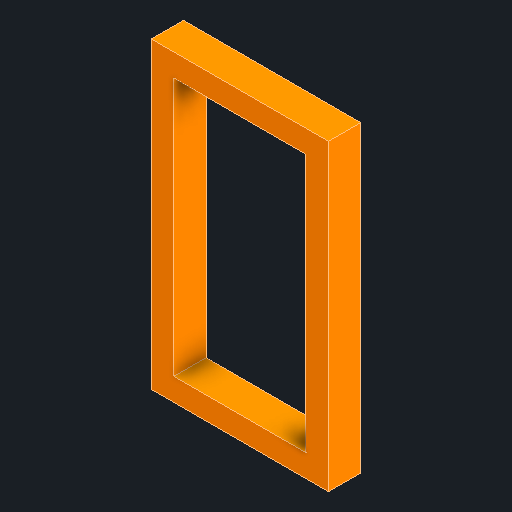
# Autodesk Inventor part: Sample Clamp
Saved by Autodesk Inventor 2023.4 (Build 274418000, 418)
## iProperties
Created: 2021-10-06
Part Number: Sample Clamp
Material: Generic
Document SubType Name: Modeling
Designer: user
Density: 1 g/cm^3
Appearance: Plastic Orange
Author: user
Autodesk Inventor part; units mm, degrees
ref_plane "YZ Plane" through (0, 0, 0) normal (1, 0, 0) x (0, 1, 0)
ref_plane "XZ Plane" through (0, 0, 0) normal (0, 1, 0) x (-1, 0, 0)
sketch "Sketch1" plane through (0, 0, 0) normal (0, 0, 1) x (1, 0, 0)
  line L0 (10, -19.8) -> (-10, -19.8) projected
  line L1 (-10, -19.8) -> (-10, -16.8) projected
  line L2 (-10, -16.8) -> (10, -16.8) projected
  line L3 (10, -16.8) -> (10, -19.8) projected
  line L4 (-10, 19.8) -> (10, 19.8) projected
  line L5 (10, 19.8) -> (10, 16.8) projected
  line L6 (10, 16.8) -> (-10, 16.8) projected
  line L7 (-10, 16.8) -> (-10, 19.8) projected
  circle A0 centre (0, 0) radius 12.5 projected
  line L8 (10, 19.8) -> (-10, 19.8)
  line L9 (-10, 19.8) -> (-10, -19.8)
  line L10 (-10, -19.8) -> (10, -19.8)
  line L11 (10, -19.8) -> (10, 19.8)
  line L12 (10.25, 20.05) -> (-10.25, 20.05)
  line L13 (-10.25, 20.05) -> (-10.25, -20.05)
  line L14 (-10.25, -20.05) -> (10.25, -20.05)
  line L15 (10.25, -20.05) -> (10.25, 20.05)
  line L16 (13.75, 23.55) -> (-13.75, 23.55)
  line L17 (-13.75, 23.55) -> (-13.75, -23.55)
  line L18 (-13.75, -23.55) -> (13.75, -23.55)
  line L19 (13.75, -23.55) -> (13.75, 23.55)
  line L20 (-20.4827, -18.7637) -> (-22.4464, -16.8) projected
  arc A1 (-18.7637, -20.4827) -> (-20.4827, -18.7637) centre (-20.5135, -20.5135) ccw projected
  line L21 (-16.8, -22.4464) -> (-18.7637, -20.4827) projected
  line L22 (-16.8, -24.65) -> (-16.8, -22.4464) projected
  line L23 (16.8, -24.65) -> (-16.8, -24.65) projected
  line L24 (16.8, -22.4464) -> (16.8, -24.65) projected
  line L25 (18.7637, -20.4827) -> (16.8, -22.4464) projected
  arc A2 (20.4827, -18.7637) -> (18.7637, -20.4827) centre (20.5135, -20.5135) ccw projected
  line L26 (22.4464, -16.8) -> (20.4827, -18.7637) projected
  line L27 (24.65, -16.8) -> (22.4464, -16.8) projected
  line L28 (24.65, 16.8) -> (24.65, -16.8) projected
  line L29 (22.4464, 16.8) -> (24.65, 16.8) projected
  line L30 (20.4827, 18.7637) -> (22.4464, 16.8) projected
  arc A3 (18.7637, 20.4827) -> (20.4827, 18.7637) centre (20.5135, 20.5135) ccw projected
  line L31 (16.8, 22.4464) -> (18.7637, 20.4827) projected
  line L32 (16.8, 24.65) -> (16.8, 22.4464) projected
  line L33 (-16.8, 24.65) -> (16.8, 24.65) projected
  line L34 (-16.8, 22.4464) -> (-16.8, 24.65) projected
  line L35 (-18.7637, 20.4827) -> (-16.8, 22.4464) projected
  arc A4 (-20.4827, 18.7637) -> (-18.7637, 20.4827) centre (-20.5135, 20.5135) ccw projected
  line L36 (-22.4464, 16.8) -> (-20.4827, 18.7637) projected
  line L37 (-24.65, 16.8) -> (-22.4464, 16.8) projected
  line L38 (-24.65, -16.8) -> (-24.65, 16.8) projected
  line L39 (-22.4464, -16.8) -> (-24.65, -16.8) projected
  point P0 (10.25, 7.1545)
  point P1 (10.25, -7.1545)
  point P2 (-10.25, -7.1545)
  point P3 (-10.25, 7.1545)
  dimension "d0" = 0.25
  dimension "d1" = 3.75
  constraints: 24 end point, 6 parallel, 3 perpendicular, 1 horizontal, 6 other
  measures "d0" distance between parallel lines of L11 L15
  measures "d1" distance between parallel lines of L11 L19
ref_plane "Work Plane1" through (-8.4, -24.65, 10.2) normal (0, 0, -1) x (-1, 0, 0)
extrude "Extrusion1" add sketch "Sketch1" along normal blind 5 from surface at 10.2 contours L15 A0 | A0 L13 | L19 L18 L17 L16
body "Solid1"
